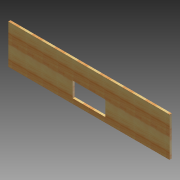
# Autodesk Inventor part: plywood back pannel
Saved by Autodesk Inventor 2012 (Build 160160000, 160)
## iProperties
Created: 2013-09-02
Part Number: plywood back pannel
Material: Default
Document SubType Name: Modeling
Designer: Bryce
Density: 1 g/cm^3
Author: Bryce
Autodesk Inventor part; units mm, degrees
ref_plane "YZ Plane" through (0, 0, 0) normal (1, 0, 0) x (0, 1, 0)
ref_plane "XZ Plane" through (0, 0, 0) normal (0, 1, 0) x (-1, 0, 0)
ref_plane "XY Plane" through (0, 0, 0) normal (0, 0, 1) x (1, 0, 0)
sketch "Sketch1" plane through (0, 0, 0) normal (0, 0, 1) x (1, 0, 0)
  line L0 (0, 0) -> (939.8, 0)
  line L1 (939.8, 0) -> (939.8, 228.6)
  line L2 (939.8, 228.6) -> (0, 228.6)
  line L3 (0, 228.6) -> (0, 0)
  line L4 (374.65, 28.575) -> (565.15, 28.575)
  line L5 (565.15, 28.575) -> (565.15, 117.475)
  line L6 (565.15, 117.475) -> (374.65, 117.475)
  line L7 (374.65, 117.475) -> (374.65, 28.575)
  dimension "d0" = 939.8
  dimension "d1" = 228.6
  dimension "d4" = 374.65
  dimension "d5" = 374.65
  dimension "d6" = 190.5
  dimension "d7" = 88.9
  dimension "d8" = 28.575
  constraints: 16 end point, 4 parallel, 2 horizontal, 2 perpendicular
  measures "d0" distance of L1.end L2.end
  measures "d1" distance of L2.end L0.start
  measures "d4" distance between parallel lines of L3 L7
  measures "d5" distance between parallel lines of L1 L5
  measures "d6" distance of L5.end L6.end
  measures "d7" distance of L6.end L4.start
  measures "d8" distance between parallel lines of L0 L4
extrude "Extrusion1" add sketch "Sketch1" along normal blind 12.7
fillet "Fillet1" radius 3.175 4 edges at (565.15, 117.475, 6.35) (374.65, 117.475, 6.35) (374.65, 28.575, 6.35) (565.15, 28.575, 6.35)
equation "\"d4\" = d5"
body "Solid1"
